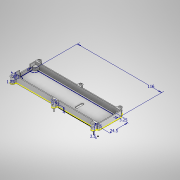
# Autodesk Inventor part: frontpack
Saved by Autodesk Inventor 2021 (Build 250183000, 183)
## iProperties
Created: 2021-09-03
Part Number: frontpack
Material: Generic
Document SubType Name: Modeling
Designer: perez
Density: 1 g/cm^3
Appearance: Default
Author: perez
Autodesk Inventor part; units mm, degrees
ref_plane "YZ Plane" through (0, 0, 0) normal (1, 0, 0) x (0, 1, 0)
ref_plane "XZ Plane" through (0, 0, 0) normal (0, 1, 0) x (-1, 0, 0)
ref_plane "XY Plane" through (0, 0, 0) normal (0, 0, 1) x (1, 0, 0)
sketch "Sketch1" plane through (0, 0, 0) normal (0, 1, 0) x (-1, 0, 0)
  line L0 (0, 0) -> (37, 0) construction
  line L1 (37, 0) -> (37, -30) construction
  line L2 (37, -30) -> (0, -30) construction
  line L3 (0, -30) -> (0, 0) construction
  line L4 (75.5, -6) -> (38, -6) construction
  line L5 (38, -6) -> (38, -24) construction
  line L6 (38, -24) -> (75.5, -24) construction
  line L7 (75.5, -24) -> (75.5, -6) construction
  line L8 (94, 0) -> (76.5, 0) construction
  line L9 (76.5, 0) -> (76.5, -28) construction
  line L10 (76.5, -28) -> (94, -28) construction
  line L11 (94, -28) -> (94, 0) construction
  line L12 (-1, 1) -> (117.5, 1)
  line L13 (117.5, 1) -> (117.5, -31)
  line L14 (117.5, -31) -> (-1, -31)
  line L15 (-1, -31) -> (-1, 1)
  line L16 (0, 0) -> (94, 0)
  line L17 (94, 0) -> (94, -30)
  line L18 (94, -30) -> (0, -30)
  line L19 (0, -30) -> (0, 0)
  line L20 (38, -8) -> (37, -8)
  line L21 (37, -8) -> (37, -22)
  line L22 (37, -22) -> (38, -22)
  line L23 (38, -22) -> (38, -8)
  line L24 (73.5, -6) -> (40, -6)
  line L25 (40, -6) -> (40, -5)
  line L26 (40, -5) -> (73.5, -5)
  line L27 (73.5, -5) -> (73.5, -6)
  line L28 (73.5, -24) -> (40, -24)
  line L29 (40, -24) -> (40, -25)
  line L30 (40, -25) -> (73.5, -25)
  line L31 (73.5, -25) -> (73.5, -24)
  line L32 (76.5, -8) -> (75.5, -8)
  line L33 (75.5, -8) -> (75.5, -22)
  line L34 (75.5, -22) -> (76.5, -22)
  line L35 (76.5, -22) -> (76.5, -8)
  line L36 (115, -31) -> (115, -33.5) construction
  line L37 (58.25, -31) -> (58.25, -33.5) construction
  line L38 (4, -31) -> (4, -33.5) construction
  line L39 (115, 1) -> (115, 3.5) construction
  line L40 (58.25, 1) -> (58.25, 3.5) construction
  line L41 (4, 1) -> (4, 3.5) construction
  circle A0 centre (115, -33.5) radius 2.5
  circle A1 centre (58.25, -33.5) radius 2.5
  circle A2 centre (4, -33.5) radius 2.5
  circle A3 centre (4, 3.5) radius 2.5
  circle A4 centre (58.25, 3.5) radius 2.5
  circle A5 centre (115, 3.5) radius 2.5
  line L42 (117.5, 1) -> (117.5, 3.5)
  line L43 (112.5, 3.5) -> (112.5, 1)
  line L44 (60.75, 3.5) -> (60.75, 1)
  line L45 (55.75, 3.5) -> (55.75, 1)
  line L46 (6.5, 3.5) -> (6.5, 1)
  line L47 (1.5, 3.5) -> (1.5, 1)
  line L48 (1.5, -33.5) -> (1.5, -31)
  line L49 (6.5, -33.5) -> (6.5, -31)
  line L50 (55.75, -33.5) -> (55.75, -31)
  line L51 (60.75, -33.5) -> (60.75, -31)
  line L52 (117.5, -33.5) -> (117.5, -31)
  line L53 (112.5, -33.5) -> (112.5, -31)
  circle A6 centre (115, -33.5) radius 1.55
  circle A7 centre (58.25, -33.5) radius 1.55
  circle A8 centre (4, -33.5) radius 1.55
  circle A9 centre (4, 3.5) radius 1.55
  circle A10 centre (58.25, 3.5) radius 1.55
  circle A11 centre (115, 3.5) radius 1.55
  line L54 (57.75, -30) -> (58.75, -30)
  line L55 (58.75, -30) -> (58.75, -25)
  line L56 (58.75, -25) -> (57.75, -25)
  line L57 (57.75, -25) -> (57.75, -30)
  line L58 (57.75, -5) -> (58.75, -5)
  line L59 (58.75, -5) -> (58.75, 0)
  line L60 (58.75, 0) -> (57.75, 0)
  line L61 (57.75, 0) -> (57.75, -5)
  line L62 (40, -25) -> (41, -25)
  line L63 (41, -25) -> (41, -30)
  line L64 (41, -30) -> (40, -30)
  line L65 (40, -30) -> (40, -25)
  line L66 (40, -5) -> (41, -5)
  line L67 (41, -5) -> (41, 0)
  line L68 (41, 0) -> (40, 0)
  line L69 (40, 0) -> (40, -5)
  line L70 (73.5, -5) -> (72.5, -5)
  line L71 (72.5, -5) -> (72.5, 0)
  line L72 (72.5, 0) -> (73.5, 0)
  line L73 (73.5, 0) -> (73.5, -5)
  line L74 (73.5, -25) -> (72.5, -25)
  line L75 (72.5, -25) -> (72.5, -30)
  line L76 (72.5, -30) -> (73.5, -30)
  line L77 (73.5, -30) -> (73.5, -25)
  dimension "d0" = 37
  dimension "d1" = 30
  dimension "d2" = 18
  dimension "d3" = 37.5
  dimension "d4" = 1
  dimension "d5" = 6
  dimension "d6" = 17.5
  dimension "d7" = 28
  dimension "d8" = 1
  dimension "d9" = 1
  dimension "d10" = 1
  dimension "d11" = 1
  dimension "d12" = 117.5
  dimension "d13" = 2
  dimension "d14" = 2
  dimension "d15" = 1
  dimension "d16" = 1
  dimension "d17" = 2
  dimension "d18" = 2
  dimension "d19" = 2
  dimension "d20" = 2
  dimension "d21" = 2.5
  dimension "d22" = 2.5
  dimension "d23" = 5
  dimension "d24" = 2.5
  dimension "d25" = 2.5
  dimension "d26" = 2.5
  dimension "d27" = 2.5
  dimension "d28" = 5
  dimension "d29" = 5
  dimension "d30" = 2.5
  dimension "d31" = 3.1
  dimension "d32" = 3.1
  dimension "d33" = 3.1
  dimension "d34" = 3.1
  dimension "d35" = 3.1
  dimension "d36" = 3.1
  dimension "d44" = 1
  dimension "d45" = 1
  dimension "d46" = 0.5
  dimension "d47" = 0
  dimension "d48" = 1
  dimension "d49" = 1
  dimension "d50" = 1
  dimension "d51" = 1
  constraints: 152 end point, 30 parallel, 24 point on line, 16 point on circle, 15 perpendicular, 14 horizontal, 12 centre point, 12 coincident, 12 vertical, 8 tangent, 22 other
  measures "d0" distance of L1.end L2.end
  measures "d1" distance of L0.end L1.end
  measures "d2" distance of L4.end L5.end
  measures "d3" distance of L5.end L6.end
  measures "d4" distance between parallel lines of L1 L5
  measures "d5" distance between parallel lines of L2 L6
  measures "d6" distance of L10.end L9.end
  measures "d7" distance of L9.end L8.end
  measures "d8" distance between parallel lines of L7 L9
  measures "d9" distance between parallel lines of L15 L3
  measures "d12" distance between parallel lines of L13 L3
  measures "d13" distance between parallel lines of L20 L4
  measures "d14" distance between parallel lines of L22 L6
  measures "d15" distance of L30.end L28.start
  measures "d16" distance of L26.end L24.start
  measures "d17" distance between parallel lines of L5 L25
  measures "d18" distance between parallel lines of L7 L27
  measures "d19" distance between parallel lines of L6 L34
  measures "d20" distance between parallel lines of L4 L32
  measures "d21" distance of L36.start L36.end
  measures "d22" distance between parallel lines of L13 L36
  measures "d23" distance between parallel lines of L15 L38
  measures "d24" distance of L37.start L37.end
  measures "d25" distance of L39.start L39.end
  measures "d26" distance of L40.start L40.end
  measures "d27" distance of L41.start L41.end
  measures "d28" diameter of A0
  measures "d29" diameter of A1
  measures "d30" distance of L38.start L38.end
  measures "d31" diameter of A6
  measures "d32" diameter of A7
  measures "d33" diameter of A8
  measures "d34" diameter of A9
  measures "d35" diameter of A10
  measures "d36" diameter of A11
  measures "d44" distance between parallel lines of L55 L57
  measures "d45" distance between parallel lines of L59 L61
  measures "d46" distance between parallel lines of L37 L57
  measures "d47" distance between parallel lines of L40 L37
  measures "d48" distance of L63.end L64.end
  measures "d49" distance of L68.end L67.end
  measures "d50" distance of L71.end L72.end
  measures "d51" distance of L76.end L75.end
extrude "Extrusion1" add sketch "Sketch1" along normal blind 7 contours L12 L13 L14 L15 | L47 A3 L12 | A3 L46 L12 | A3 | L14 A2 L48 | L14 L49 A2 | A2 | L45 A4 L12 | A4 L44 L12 | A4 | L14 A1 L50 | L14 L51 A1 | A1 | L43 A5 L12 | A5 L42 L12 | A5 | L14 A0 L53 | L14 L52 A0 | A0 | L16 L67 L26 L69 | L26 L27 L24 L25 | L65 L30 L63 L18 | L16 L59 L26 L61 | L29 L28 L31 L30 | L57 L30 L55 L18 | L16 L73 L26 L71 | L75 L30 L77 L18 | L23 L22 L21 L20 | L35 L34 L33 L32
sketch "Sketch2" plane through (0, 0, 0) normal (0, -1, 0) x (1, 0, 0)
  line L0 (-117.5, -33.5) -> (-117.5, 3.5) projected
  arc A0 (-117.5, -33.5) -> (-112.5, -33.5) centre (-115, -33.5) ccw projected
  line L1 (-112.5, -31) -> (-112.5, -33.5) projected
  line L2 (-60.75, -31) -> (-112.5, -31) projected
  line L3 (-60.75, -33.5) -> (-60.75, -31) projected
  arc A1 (-60.75, -33.5) -> (-55.75, -33.5) centre (-58.25, -33.5) ccw projected
  line L4 (-55.75, -31) -> (-55.75, -33.5) projected
  line L5 (-6.5, -31) -> (-55.75, -31) projected
  line L6 (-6.5, -33.5) -> (-6.5, -31) projected
  arc A2 (-6.5, -33.5) -> (-1.5, -33.5) centre (-4, -33.5) ccw projected
  line L7 (-1.5, -31) -> (-1.5, -33.5) projected
  line L8 (1, -31) -> (-1.5, -31) projected
  line L9 (1, 1) -> (1, -31) projected
  line L10 (-1.5, 1) -> (1, 1) projected
  line L11 (-1.5, 3.5) -> (-1.5, 1) projected
  arc A3 (-1.5, 3.5) -> (-6.5, 3.5) centre (-4, 3.5) ccw projected
  line L12 (-6.5, 1) -> (-6.5, 3.5) projected
  line L13 (-55.75, 1) -> (-6.5, 1) projected
  line L14 (-55.75, 3.5) -> (-55.75, 1) projected
  arc A4 (-55.75, 3.5) -> (-60.75, 3.5) centre (-58.25, 3.5) ccw projected
  line L15 (-60.75, 1) -> (-60.75, 3.5) projected
  line L16 (-112.5, 1) -> (-60.75, 1) projected
  line L17 (-112.5, 3.5) -> (-112.5, 1) projected
  arc A5 (-112.5, 3.5) -> (-117.5, 3.5) centre (-115, 3.5) ccw projected
  circle A6 centre (-58.25, 3.5) radius 1.55 projected
  circle A7 centre (-4, 3.5) radius 1.55 projected
  circle A8 centre (-4, -33.5) radius 1.55 projected
  circle A9 centre (-58.25, -33.5) radius 1.55 projected
  circle A10 centre (-115, 3.5) radius 1.55 projected
  circle A11 centre (-115, -33.5) radius 1.55 projected
  line L18 (-41, 0) -> (-57.75, 0) projected
  line L19 (0, -30) -> (0, 0) projected
  line L20 (-57.75, -30) -> (-41, -30) projected
  line L21 (-94, 0) -> (-94, -30) projected
  line L22 (-41, -5) -> (-41, 0) projected
  line L23 (-57.75, -5) -> (-41, -5) projected
  line L24 (-57.75, 0) -> (-57.75, -5) projected
  line L25 (-41, -30) -> (-41, -25) projected
  line L26 (-57.75, -25) -> (-57.75, -30) projected
  line L27 (-41, -25) -> (-57.75, -25) projected
  line L28 (-72.5, -25) -> (-72.5, -30) projected
  line L29 (-58.75, -25) -> (-72.5, -25) projected
  line L30 (-58.75, -30) -> (-58.75, -25) projected
  line L31 (-72.5, -30) -> (-58.75, -30) projected
  line L32 (-72.5, 0) -> (-72.5, -5) projected
  line L33 (-58.75, 0) -> (-72.5, 0) projected
  line L34 (-58.75, -5) -> (-58.75, 0) projected
  line L35 (-72.5, -5) -> (-58.75, -5) projected
  line L36 (-73.5, 0) -> (-94, 0) projected
  line L37 (-73.5, -6) -> (-73.5, 0) projected
  line L38 (-40, -6) -> (-73.5, -6) projected
  line L39 (-40, 0) -> (-40, -6) projected
  line L40 (0, 0) -> (-40, 0) projected
  line L41 (-40, -30) -> (0, -30) projected
  line L42 (-40, -24) -> (-40, -30) projected
  line L43 (-73.5, -24) -> (-40, -24) projected
  line L44 (-73.5, -30) -> (-73.5, -24) projected
  line L45 (-94, -30) -> (-73.5, -30) projected
extrude "Extrusion2" add sketch "Sketch2" along normal blind 1 contours L0 A5 L17 L16 L15 A4 L14 L13 L12 A3 L11 L10 L9 L8 L7 A2 L6 L5 L4 A1 L3 L2 L1 A0 | L22 L23 L24 L18 | L41 L42 L43 L44 L45 L21 L36 L37 L38 L39 L40 L19 | L26 L27 L25 L20 | L29 L30 L31 L28 | L33 L34 L35 L32
fillet "Fillet2" radius 1 32 edges at (-73.5, 3.5, -6) (-73.5, 3.5, -24) (-40, 3.5, -24) (1, 3, -31) (-1.5, 3, -31) (1, 3, 1) (-55.75, 3, -31) (-1.5, 3, 1) (-55.75, 3, 1) (-112.5, 3, 1) (-112.5, 3, -31) (-60.75, 3, -31) (-6.5, 3, -31) (-60.75, 3, 1) (-6.5, 3, 1) (-40, 3.5, -6) (-72.5, 3.5, 0) (-57.75, 3.5, 0) (-72.5, 3.5, -25) (-57.75, 3.5, -25) (-41, 3.5, -25) (-58.75, 3.5, -25) (-41, 3.5, 0) (-58.75, 3.5, 0) (-72.5, 3.5, -30) (-57.75, 3.5, -30) (-57.75, 3.5, -5) (-72.5, 3.5, -5) (-41, 3.5, -5) (-58.75, 3.5, -5) (-58.75, 3.5, -30) (-41, 3.5, -30)
sketch "Sketch5" plane through (0, 7, 0) normal (0, 1, 0) x (1, 0, 0)
  line L0 (-120.447, 38.9055) -> (3.6698, 38.9055)
  line L1 (3.6698, 38.9055) -> (3.6698, -10.7705)
  line L2 (3.6698, -10.7705) -> (-120.447, -10.7705)
  line L3 (-120.447, -10.7705) -> (-120.447, 38.9055)
  point P0 (0, 0)
  constraints: 8 end point, 2 parallel, 1 horizontal, 1 perpendicular
extrude "Extrusion5" cut sketch "Sketch5" against normal blind 7
sketch "Sketch6" plane through (0, 0, 0) normal (0, 1, 0) x (1, 0, 0)
  line L0 (-116.25, 27.75) -> (-0.25, 27.75)
  line L1 (-0.25, 27.75) -> (-0.25, 3.25)
  line L2 (-0.25, 3.25) -> (-116.25, 3.25)
  line L3 (-116.25, 3.25) -> (-116.25, 27.75)
  line L4 (-117.5, -3.5) -> (-117.5, 33.5) projected
  line L5 (-54.75, 31) -> (-7.5, 31) projected
  line L6 (-117.5, 9.25) -> (-116.25, 9.25)
  line L7 (-116.25, 9.25) -> (-116.25, 3.25)
  line L8 (-116.25, 3.25) -> (-117.5, 3.25)
  line L9 (-117.5, 3.25) -> (-117.5, 9.25)
  circle A0 centre (-58.25, -3.5) radius 1.55 projected
  circle A1 centre (-4, -3.5) radius 1.55 projected
  circle A2 centre (-4, 33.5) radius 1.55 projected
  circle A3 centre (-58.25, 33.5) radius 1.55 projected
  circle A4 centre (-115, -3.5) radius 1.55 projected
  circle A5 centre (-115, 33.5) radius 1.55 projected
  arc A6 (1, 30) -> (0, 31) centre (0, 30) ccw projected
  line L10 (-0.5, 31) -> (0, 31) projected
  arc A7 (-1.5, 32) -> (-0.5, 31) centre (-0.5, 32) ccw projected
  line L11 (-1.5, 33.5) -> (-1.5, 32) projected
  arc A8 (-1.5, 33.5) -> (-6.5, 33.5) centre (-4, 33.5) ccw projected
  line L12 (-6.5, 32) -> (-6.5, 33.5) projected
  arc A9 (-7.5, 31) -> (-6.5, 32) centre (-7.5, 32) ccw projected
  line L13 (-54.75, 31) -> (-7.5, 31) projected
  arc A10 (-55.75, 32) -> (-54.75, 31) centre (-54.75, 32) ccw projected
  line L14 (-55.75, 33.5) -> (-55.75, 32) projected
  arc A11 (-55.75, 33.5) -> (-60.75, 33.5) centre (-58.25, 33.5) ccw projected
  line L15 (-60.75, 32) -> (-60.75, 33.5) projected
  arc A12 (-61.75, 31) -> (-60.75, 32) centre (-61.75, 32) ccw projected
  line L16 (-111.5, 31) -> (-61.75, 31) projected
  arc A13 (-112.5, 32) -> (-111.5, 31) centre (-111.5, 32) ccw projected
  line L17 (-112.5, 33.5) -> (-112.5, 32) projected
  arc A14 (-112.5, 33.5) -> (-117.5, 33.5) centre (-115, 33.5) ccw projected
  line L18 (-117.5, -3.5) -> (-117.5, 33.5) projected
  arc A15 (-117.5, -3.5) -> (-112.5, -3.5) centre (-115, -3.5) ccw projected
  line L19 (-112.5, -2) -> (-112.5, -3.5) projected
  arc A16 (-111.5, -1) -> (-112.5, -2) centre (-111.5, -2) ccw projected
  line L20 (-61.75, -1) -> (-111.5, -1) projected
  arc A17 (-60.75, -2) -> (-61.75, -1) centre (-61.75, -2) ccw projected
  line L21 (-60.75, -3.5) -> (-60.75, -2) projected
  arc A18 (-60.75, -3.5) -> (-55.75, -3.5) centre (-58.25, -3.5) ccw projected
  line L22 (-55.75, -2) -> (-55.75, -3.5) projected
  arc A19 (-54.75, -1) -> (-55.75, -2) centre (-54.75, -2) ccw projected
  line L23 (-7.5, -1) -> (-54.75, -1) projected
  arc A20 (-6.5, -2) -> (-7.5, -1) centre (-7.5, -2) ccw projected
  line L24 (-6.5, -3.5) -> (-6.5, -2) projected
  arc A21 (-6.5, -3.5) -> (-1.5, -3.5) centre (-4, -3.5) ccw projected
  line L25 (-1.5, -2) -> (-1.5, -3.5) projected
  arc A22 (-0.5, -1) -> (-1.5, -2) centre (-0.5, -2) ccw projected
  line L26 (0, -1) -> (-0.5, -1) projected
  arc A23 (0, -1) -> (1, 0) centre (0, 0) ccw projected
  line L27 (1, 30) -> (1, 0) projected
  line L28 (-116.25, 27.75) -> (-117.5, 27.75)
  line L29 (-117.5, 27.75) -> (-117.5, 21.75)
  line L30 (-117.5, 21.75) -> (-116.25, 21.75)
  line L31 (-116.25, 21.75) -> (-116.25, 27.75)
  arc A24 (-110.25, 3.25) -> (-116.25, 9.25) centre (-116.25, 3.25) ccw
  arc A25 (-116.25, 21.75) -> (-110.25, 27.75) centre (-116.25, 27.75) ccw
  arc A26 (-5.25, 27.75) -> (-0.25, 22.75) centre (-0.25, 27.75) ccw
  arc A27 (-0.25, 8.25) -> (-5.25, 3.25) centre (-0.25, 3.25) ccw
  point P0 (0, 0)
  point P1 (-7.5, 31)
  dimension "d63" = 24.5
  dimension "d64" = 116
  dimension "d65" = 1.25
  dimension "d66" = 3.25
  dimension "d67" = 6
  dimension "d68" = 6
  dimension "d71" = 5
  dimension "d72" = 5
  constraints: 24 end point, 8 point on circle, 8 point on line, 6 parallel, 4 centre point, 4 coincident, 3 horizontal, 3 perpendicular
  measures "d63" distance between parallel lines of L2 L0
  measures "d64" distance of L0.start L0.end
  measures "d65" distance between parallel lines of L4 L3
  measures "d66" distance between parallel lines of L5 L0
  measures "d67" distance between parallel lines of L8 L6
  measures "d68" distance between parallel lines of L30 L28
  measures "d71" radius of A26
  measures "d72" radius of A27
extrude "Extrusion6" add sketch "Sketch6" along normal blind 4 contours L28 L4 A14 L17 A13 L16 A12 L15 A11 L14 A10 L5 A9 L12 A8 L11 A7 L10 A6 L27 A23 L26 A22 L25 A21 L24 A20 L23 A19 L22 A18 L21 A17 L20 A16 L19 A15 L8 L2 L1 L0 | L0 A25 L3 | L3 L30 L4 L28 | L3 L6 L4 L30 | L0 L1 A26 | A24 L2 L3 | L3 L8 L4 L6 | L1 L2 A27
extrude "Extrusion7" add sketch "Sketch6" along normal blind 3.5 from surface at 4 contours L28 L4 A14 L17 A13 L16 A12 L15 A11 L14 A10 L5 A9 L12 A8 L11 A7 L10 A6 L27 A23 L26 A22 L25 A21 L24 A20 L23 A19 L22 A18 L21 A17 L20 A16 L19 A15 L8 L2 L1 L0 | L3 L30 L4 L28 | L3 L8 L4 L6
sketch "Sketch7" plane through (0, 0, 0) normal (0, 1, 0) x (1, 0, 0)
  arc A0 (-42.63, 11.1) -> (-39.6307, 11.1465) centre (-41.13, 11.1) ccw
  arc A1 (-39.63, 18.8999) -> (-42.63, 18.9) centre (-41.13, 18.9) ccw
  line L0 (-38, 8) -> (-38, 22)
  line L1 (-41, 6) -> (-72.5, 6)
  line L2 (-72.5, 24) -> (-41, 24)
  line L3 (-39.6307, 11.0533) -> (-39.63, 18.8999)
  line L4 (-42.63, 11.1) -> (-42.63, 18.9)
  line L5 (1, 30) -> (1, 0) projected
  point P0 (0, 0)
  point P1 (0, 0)
  dimension "d75" = 3
  dimension "d76" = 3
  dimension "d77" = 3.13
  dimension "d78" = 5.1
  dimension "d79" = 5.1
  dimension "d80" = 0
  dimension "d81" = 42.13
  constraints: 10 end point, 5 point on circle, 2 centre point, 2 tangent, 1 point on line
  measures "d75" diameter of A0
  measures "d76" diameter of A1
  measures "d77" distance from line of L0 A0.centre
  measures "d78" distance from line of L1 A0.centre
  measures "d79" distance from line of L2 A1.centre
  measures "d80" horizontal distance of A0.centre A1.centre
  measures "d81" distance from line of L5 A0.centre
extrude "Extrusion8" cut sketch "Sketch7" against normal through all
sketch "Sketch8" plane through (-54.75, -1, 1) normal (0, 0, 1) x (1, 0, 0)
  circle A0 centre (-3.5267, 4) radius 1
  circle A1 centre (50.75, 4) radius 1
  line L0 (0, 0) -> (47.25, 0)
  line L1 (-6, -8) -> (-6.0178, 0)
  line L2 (48.25, -8) -> (48.25, 0)
  line L3 (-6, 0) -> (-1, 0) projected
  circle A2 centre (-60.25, 4) radius 1
  line L4 (-62.75, 0) -> (-62.75, 8.5) projected
  point P0 (54.75, 1)
  point P1 (54.75, -7)
  dimension "d84" = 2
  dimension "d85" = 2
  dimension "d87" = 2.5
  dimension "d88" = 2.5
  dimension "d89" = 4
  dimension "d92" = 2
  dimension "d93" = 2.5
  constraints: 6 end point, 3 centre point, 1 horizontal alignment
  measures "d84" diameter of A0
  measures "d85" diameter of A1
  measures "d87" distance from line of L1 A0.centre
  measures "d88" distance from line of L2 A1.centre
  measures "d89" distance from line of L3 A0.centre
  measures "d92" diameter of A2
  measures "d93" distance from line of L4 A2.centre
extrude "Extrusion9" cut sketch "Sketch8" along normal blind 10
extrude "Extrusion10" cut sketch "Sketch8" against normal blind 20 from surface at -32
sketch "Sketch9" plane through (-116.25, 7.5, -27.75) normal (0, 1, 0) x (1, 0, 0)
  line L0 (-0.25, -27.75) -> (116.25, -27.75)
  line L1 (116.25, -27.75) -> (116.25, 2.25)
  line L2 (116.25, 2.25) -> (-0.25, 2.25)
  line L3 (-0.25, 2.25) -> (-0.25, -27.75)
  line L4 (4.75, 3.25) -> (54.5, 3.25) projected
  line L5 (-1.25, -6) -> (-1.25, -18.5) projected
  dimension "d96" = 30
  dimension "d97" = 1
  dimension "d100" = 116.5
  dimension "d101" = 1
  constraints: 8 end point, 2 parallel, 1 horizontal, 1 perpendicular
  measures "d96" distance between parallel lines of L2 L0
  measures "d97" distance between parallel lines of L2 L4
  measures "d100" distance of L1.end L2.end
  measures "d101" distance between parallel lines of L3 L5
extrude "Extrusion11" cut sketch "Sketch9" against normal up to surface (3.5 mm away)
sketch "Sketch10" plane through (0, 4, 0) normal (0, 1, 0) x (1, 0, 0)
  line L0 (-116.5, 0) -> (-116.5, 9.25) projected
  line L1 (0, 0) -> (-116.5, 0) projected
  line L2 (0, 30) -> (0, 0) projected
  line L3 (-116.5, 30) -> (0, 30) projected
  line L4 (-116.5, 21.75) -> (-116.5, 30) projected
  line L5 (-116.5, 21.75) -> (-117.5, 21.75) projected
  line L6 (-117.5, 21.75) -> (-117.5, 9.25) projected
  line L7 (-117.5, 9.25) -> (-116.5, 9.25) projected
  arc A0 (-110.25, 3.25) -> (-116.25, 9.25) centre (-116.25, 3.25) ccw projected
  line L8 (-116.25, 9.25) -> (-116.25, 21.75) projected
  arc A1 (-116.25, 21.75) -> (-110.25, 27.75) centre (-116.25, 27.75) ccw projected
  line L9 (-5.25, 27.75) -> (-110.25, 27.75) projected
  arc A2 (-5.25, 27.75) -> (-0.25, 22.75) centre (-0.25, 27.75) ccw projected
  line L10 (-0.25, 8.25) -> (-0.25, 22.75) projected
  arc A3 (-0.25, 8.25) -> (-5.25, 3.25) centre (-0.25, 3.25) ccw projected
  line L11 (-110.25, 3.25) -> (-5.25, 3.25) projected
  line L12 (-116.5, 30) -> (0, 30) projected
  arc A4 (-5, 30) -> (0, 25) centre (0, 30) ccw
  line L13 (0, 30) -> (0, 0) projected
  line L14 (0, 0) -> (-116.5, 0) projected
  arc A5 (0, 5) -> (-5, 0) centre (0, 0) ccw
  arc A6 (-111.5, 0) -> (-116.5, 5) centre (-116.5, 0) ccw
  line L15 (-116.5, 21.75) -> (-116.5, 30) projected
  arc A7 (-116.5, 25) -> (-111.5, 30) centre (-116.5, 30) ccw
  point P0 (-5, 0)
  point P1 (-116.5, 25)
  dimension "d102" = 5
  dimension "d103" = 5
  dimension "d104" = 5
  dimension "d105" = 5
  constraints: 8 point on circle, 7 point on line, 4 centre point, 4 coincident
  measures "d102" radius of A4
  measures "d103" radius of A5
  measures "d104" radius of A6
  measures "d105" radius of A7
extrude "Extrusion12" cut sketch "Sketch10" against normal up to surface (4 mm away) contours L0 L7 L6 L5 L4 A7 L3 A4 L2 A5 L1 A6
sketch "Sketch11" plane through (0, 0, 0) normal (0, 1, 0) x (1, 0, 0)
  line L0 (-116.5, 21.75) -> (-117.5, 21.75) projected
  line L1 (-117.5, 9.25) -> (-116.5, 9.25) projected
  line L2 (-117.5, 21.75) -> (-116.5, 21.75)
  line L3 (-116.5, 21.75) -> (-116.5, 9.25)
  line L4 (-116.5, 9.25) -> (-117.5, 9.25)
  line L5 (-117.5, 9.25) -> (-117.5, 21.75)
  point P0 (0, 0)
  constraints: 8 end point, 2 parallel, 1 horizontal, 1 perpendicular
extrude "Extrusion13" add sketch "Sketch6" along normal up to surface (4 mm away) contours L3 L6 L4 L30
sketch "Sketch12" plane through (-111.5, 7.5, 1) normal (0, 1, 0) x (1, 0, 0)
  line L0 (-6, 22.75) -> (-6, 34.5) projected
  line L1 (-5, 1) -> (-5, 10.25) projected
  line L2 (-6, 23.75) -> (-5, 23.75)
  line L3 (-5, 23.75) -> (-5, 9.25)
  line L4 (-5, 9.25) -> (-6, 9.25)
  line L5 (-6, 9.25) -> (-6, 23.75)
  line L6 (-5, 22.75) -> (-6, 22.75) projected
  line L7 (-6, 10.25) -> (-5, 10.25) projected
  point P0 (111.5, 1)
  dimension "d110" = 1
  dimension "d111" = 1
  constraints: 8 end point, 2 parallel, 2 point on line, 1 horizontal, 1 perpendicular
  measures "d110" distance between parallel lines of L6 L2
  measures "d111" distance between parallel lines of L7 L4
extrude "Extrusion14" cut sketch "Sketch12" against normal up to surface (3.5 mm away)
body "Solid1"
